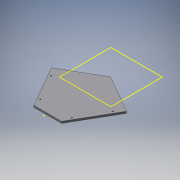
# Autodesk Inventor part: bottom top plate
Saved by Autodesk Inventor 2016 SP1 (Build 200210100, 210)
## iProperties
Created: 2016-04-14
Part Number: bottom top plate
Material: Generic
Document SubType Name: Modeling
Designer: ubik
Density: 1 g/cm^3
Appearance: Default
Author: ubik
Autodesk Inventor part; units mm, degrees
ref_plane "YZ Plane" through (0, 0, 0) normal (1, 0, 0) x (0, 1, 0)
ref_plane "XZ Plane" through (0, 0, 0) normal (0, 1, 0) x (-1, 0, 0)
ref_plane "XY Plane" through (0, 0, 0) normal (0, 0, 1) x (1, 0, 0)
sketch "Sketch1" plane through (0, 0, 0) normal (0, 0, 1) x (1, 0, 0)
  arc A0 (-16.5011, 13.8506) -> (-21.6973, 4.8506) centre (-16.5011, 7.8506) ccw projected
  line L0 (-16.5011, 13.8506) -> (16.5011, 13.8506) projected
  arc A1 (21.6973, 4.8506) -> (16.5011, 13.8506) centre (16.5011, 7.8506) ccw projected
  line L1 (21.6973, 4.8506) -> (13.3257, -9.6494) projected
  arc A2 (5.5315, -14.1494) -> (13.3257, -9.6494) centre (5.5315, -5.1494) ccw projected
  line L2 (5.5315, -14.1494) -> (-5.5315, -14.1494) projected
  arc A3 (-13.3257, -9.6494) -> (-5.5315, -14.1494) centre (-5.5315, -5.1494) ccw projected
  line L3 (-13.3257, -9.6494) -> (-21.6973, 4.8506) projected
  line L4 (10, -20.5494) -> (10, -40.5494) projected
  line L5 (10, -40.5494) -> (-10, -40.5494) projected
  line L6 (-10, -40.5494) -> (-10, -20.5494) projected
  line L7 (-10, -20.5494) -> (10, -20.5494) projected
  line L8 (-15, -16.7494) -> (-32.2735, -26.7222) projected
  arc A4 (-32.2735, -26.7222) -> (32.2735, -26.7222) centre (0, -5.7301) ccw projected
  line L9 (32.2735, -26.7222) -> (15, -16.7494) projected
  line L10 (23.4871, 17.4506) -> (-23.4871, 17.4506)
  arc A5 (-222.749, 428.2443) -> (-227.9452, 437.2443) centre (-227.9452, 431.2443) ccw projected
  line L11 (-222.749, 428.2443) -> (-239.2501, 399.6635) projected
  arc A6 (-249.6424, 399.6635) -> (-239.2501, 399.6635) centre (-244.4463, 402.6635) ccw projected
  line L12 (-249.6424, 399.6635) -> (-258.014, 414.1635) projected
  arc A7 (-258.014, 423.1635) -> (-258.014, 414.1635) centre (-250.2198, 418.6635) ccw projected
  line L13 (-258.014, 423.1635) -> (-252.4825, 432.7443) projected
  arc A8 (-244.6883, 437.2443) -> (-252.4825, 432.7443) centre (-244.6883, 428.2443) ccw projected
  line L14 (-244.6883, 437.2443) -> (-227.9452, 437.2443) projected
  line L15 (-265.7908, 422.4937) -> (-283.1113, 432.4937) projected
  line L16 (-283.1113, 432.4937) -> (-273.1113, 449.8142) projected
  line L17 (-273.1113, 449.8142) -> (-255.7908, 439.8142) projected
  line L18 (-255.7908, 439.8142) -> (-265.7908, 422.4937) projected
  line L19 (-193.9999, 442.2443) -> (-249.9999, 442.2443) projected
  line L20 (-249.9999, 442.2443) -> (-249.9999, 462.19) projected
  arc A9 (-249.9999, 462.19) -> (-282.2735, 406.2907) centre (-247.957, 423.7443) ccw projected
  line L21 (-282.2735, 406.2907) -> (-264.9999, 416.2635) projected
  line L22 (-264.9999, 416.2635) -> (-237, 367.7661) projected
  line L23 (-237, 367.7661) -> (-232.6699, 370.2661) projected
  line L24 (-232.6699, 370.2661) -> (-239.6254, 382.3135) projected
  arc A10 (-239.6254, 391.8135) -> (-239.6254, 382.3135) centre (-231.3982, 387.0635) ccw projected
  line L25 (-239.6254, 391.8135) -> (-216.1383, 432.4943) projected
  arc A11 (-207.9111, 437.2443) -> (-216.1383, 432.4943) centre (-207.9111, 427.7443) ccw projected
  line L26 (-207.9111, 437.2443) -> (-193.9999, 437.2443) projected
  line L27 (-193.9999, 437.2443) -> (-193.9999, 442.2443) projected
  arc A12 (239.2502, 399.6633) -> (249.6425, 399.6633) centre (244.4464, 402.6633) ccw projected
  line L28 (239.2502, 399.6633) -> (222.7491, 428.2441) projected
  arc A13 (227.9453, 437.2441) -> (222.7491, 428.2441) centre (227.9453, 431.2441) ccw projected
  line L29 (227.9453, 437.2441) -> (244.6884, 437.2441) projected
  arc A14 (252.4827, 432.7441) -> (244.6884, 437.2441) centre (244.6884, 428.2441) ccw projected
  line L30 (252.4827, 432.7441) -> (258.0141, 423.1633) projected
  arc A15 (258.0141, 414.1633) -> (258.0141, 423.1633) centre (250.2199, 418.6633) ccw projected
  line L31 (258.0141, 414.1633) -> (249.6425, 399.6633) projected
  line L32 (255.791, 439.8139) -> (273.1115, 449.8139) projected
  line L33 (273.1115, 449.8139) -> (283.1115, 432.4934) projected
  line L34 (283.1115, 432.4934) -> (265.791, 422.4934) projected
  line L35 (265.791, 422.4934) -> (255.791, 439.8139) projected
  line L36 (237.0001, 367.7659) -> (265.0001, 416.2633) projected
  line L37 (265.0001, 416.2633) -> (282.2736, 406.2904) projected
  arc A16 (282.2736, 406.2904) -> (250.0001, 462.1898) centre (247.9571, 423.7441) ccw projected
  line L38 (250.0001, 462.1898) -> (250.0001, 442.2441) projected
  line L39 (250.0001, 442.2441) -> (194.0001, 442.2441) projected
  line L40 (194.0001, 442.2441) -> (194.0001, 437.2441) projected
  line L41 (194.0001, 437.2441) -> (207.9112, 437.2441) projected
  arc A17 (216.1385, 432.4941) -> (207.9112, 437.2441) centre (207.9112, 427.7441) ccw projected
  line L42 (216.1385, 432.4941) -> (239.6255, 391.8133) projected
  arc A18 (239.6255, 382.3133) -> (239.6255, 391.8133) centre (231.3983, 387.0633) ccw projected
  line L43 (239.6255, 382.3133) -> (232.6699, 370.2659) projected
  line L44 (232.6699, 370.2659) -> (237.0001, 367.7659) projected
  line L45 (-249.9999, 462.19) -> (250.0001, 462.1898)
  line L46 (282.2736, 406.2904) -> (32.2735, -26.7222)
  line L47 (-32.2735, -26.7222) -> (-282.2735, 406.2907)
  line L48 (-23.4871, 17.4506) -> (-57.7767, 17.4506)
  line L49 (23.4871, 17.4506) -> (57.7768, 17.4506)
  line L50 (0, 0) -> (0, 280.5861)
  line L51 (-247.957, 423.7443) -> (0, 280.5861)
  line L52 (247.9571, 423.7441) -> (0, 280.5861)
  line L53 (0, 280.5861) -> (-157.2735, 189.7842)
  line L54 (0, 280.5861) -> (157.2736, 189.7841)
  line L55 (0, 280.5861) -> (0.0001, 462.1899)
  circle A19 centre (-128.6133, 160.1432) radius 2.5
  circle A20 centre (-66.1133, 51.89) radius 2.5
  circle A21 centre (66.1133, 51.8899) radius 2.5
  circle A22 centre (128.6133, 160.1431) radius 2.5
  dimension "d0" = 5
  dimension "d1" = 5
  dimension "d2" = 5
  dimension "d3" = 5
  dimension "d4" = 10
  dimension "d5" = 10
  dimension "d6" = 10
  dimension "d7" = 10
  dimension "d8" = 40
  dimension "d9" = 40
  dimension "d10" = 125
  dimension "d11" = 125
  constraints: 24 end point, 4 centre point, 4 point on line, 3 midpoint, 1 horizontal
  measures "d0" diameter of A19
  measures "d1" diameter of A20
  measures "d2" diameter of A21
  measures "d3" diameter of A22
  measures "d4" distance from line of L47 A19.centre
  measures "d5" distance from line of L47 A20.centre
  measures "d6" distance from line of L46 A22.centre
  measures "d7" distance from line of L46 A21.centre
  measures "d8" distance from line of L53 A19.centre
  measures "d9" distance from line of L54 A22.centre
  measures "d10" distance of A22.centre A21.centre
  measures "d11" distance of A20.centre A19.centre
extrude "Extrusion1" add sketch "Sketch1" along normal blind 8 contours L47 L53 L50 L10 L48 | L49 L10 L50 L54 L46
sketch "Sketch2" plane through (0, 0, 8) normal (0, 0, 1) x (1, 0, 0)
  line L0 (-107.5, 173.0861) -> (107.5, 173.0861) projected
  line L1 (107.5, 173.0861) -> (107.5, 388.0861) projected
  line L2 (107.5, 388.0861) -> (-107.5, 388.0861) projected
  line L3 (-107.5, 388.0861) -> (-107.5, 173.0861) projected
  point P0 (0, 0)
extrude "Extrusion2" cut sketch "Sketch2" against normal blind 3
equation "\"d5\" = d4"
equation "\"d6\" = d4"
equation "\"d7\" = d6"
equation "\"d9\" = d8"
equation "\"d11\" = d10"
body "Solid1"
